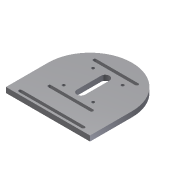
# Autodesk Inventor part: JointB1
Saved by Autodesk Inventor 2013 (Build 170138000, 138)
## iProperties
Created: 2012-10-15
Part Number: JointB1
Document SubType Name: Modeling
Designer: JohnHenry
Density: 1 g/cm^3
Mass: 25.0658 g
Surface Area: 135.276 cm^2
Volume: 25.0658 cm^3
Material: 一般
Author: JohnHenry
Autodesk Inventor part; units mm, degrees
ref_plane "YZ Plane" through (0, 0, 0) normal (1, 0, 0) x (0, 1, 0)
ref_plane "XZ Plane" through (0, 0, 0) normal (0, 1, 0) x (-1, 0, 0)
ref_plane "XY Plane" through (0, 0, 0) normal (0, 0, 1) x (1, 0, 0)
sketch "スケッチ1" plane through (0, 0, 0) normal (0, 0, 1) x (1, 0, 0)
  line L0 (-40, 67.6823) -> (40, 67.6823)
  line L1 (40, 67.6823) -> (40, -12.3177)
  line L2 (40, -12.3177) -> (-40, -12.3177)
  line L3 (-40, -12.3177) -> (-40, 67.6823)
  point P0 (0, 0)
  dimension "d0" = 80
  dimension "d1" = 40
  dimension "d2" = 80
  constraints: 8 end point, 2 parallel, 1 horizontal, 1 perpendicular
  measures "d0" distance of L1.end L2.end
  measures "d1" distance from line of L3 point (0, 0)
  measures "d2" distance of L2.end L0.start
extrude "押し出し1" add sketch "スケッチ1" along normal blind 5
sketch "スケッチ5" plane through (0, 0, 5) normal (0, 0, 1) x (1, 0, 0)
  line L0 (-40, -7.3177) -> (40, -7.3177) projected
  line L1 (40, 67.6823) -> (40, -12.3177) projected
  line L2 (-40, 67.6823) -> (40, 67.6823) projected
  line L3 (-40, -12.3177) -> (-40, 67.6823) projected
  arc A0 (40, 27.6823) -> (-40, 27.6823) centre (0, 27.6823) ccw
  point P0 (0, 0)
  dimension "d21" = 40
  dimension "d22" = 40
  dimension "d23" = 80
  constraints: 2 midpoint, 2 point on circle, 1 centre point, 1 coincident
  measures "d21" distance from line of point (0, 27.682) L2
  measures "d22" distance from line of L3 point (0, 27.682)
  measures "d23" diameter of A0
extrude "押し出し4" cut sketch "スケッチ5" against normal through all contours L3 L2 A0 | A0 L2 L1
sketch "スケッチ6" plane through (0, 0, 5) normal (0, 0, 1) x (1, 0, 0)
  arc A0 (40, 27.6823) -> (-40, 27.6823) centre (0, 27.6823) ccw projected
  point P0 (0, 0)
  constraints: 1 coincident
hole "Hole2" at (0, 27.6823, 5) direction (0, 0, -1) diameter 8 end through all
sketch "スケッチ8" plane through (0, 0, 5) normal (0, 0, 1) x (1, 0, 0)
  circle A0 centre (0, 27.6823) radius 4 projected
  line L0 (-20, 10.6823) -> (20, 10.6823)
  line L1 (20, 10.6823) -> (20, 7.6823)
  line L2 (20, 7.6823) -> (-20, 7.6823)
  line L3 (-20, 7.6823) -> (-20, 10.6823)
  circle A1 centre (-20, 9.1823) radius 1.5
  circle A2 centre (20, 9.1823) radius 1.5
  line L4 (40, -12.3177) -> (-40, -12.3177) projected
  line L5 (-20, 53.6823) -> (20, 53.6823)
  line L6 (20, 53.6823) -> (20, 50.6823)
  line L7 (20, 50.6823) -> (-20, 50.6823)
  line L8 (-20, 50.6823) -> (-20, 53.6823)
  circle A3 centre (-20, 52.1823) radius 1.5
  circle A4 centre (20, 52.1823) radius 1.5
  point P0 (0, 0)
  dimension "d54" = 3
  dimension "d55" = 20
  dimension "d56" = 40
  dimension "d65" = 20
  dimension "d87" = 40
  dimension "d88" = 20
  dimension "d89" = 3
  dimension "d91" = 40
  constraints: 16 end point, 4 midpoint, 4 parallel, 4 vertical alignment, 2 horizontal, 2 perpendicular, 8 other
  measures "d54" distance of L0.end L1.end
  measures "d55" distance from line of A0.centre L1
  measures "d56" distance of L1.end L2.end
  measures "d65" distance between parallel lines of L4 L2
  measures "d87" distance of L5.start L5.end
  measures "d88" distance from line of A0.centre L6
  measures "d89" distance of L5.end L6.end
  measures "d91" distance between parallel lines of L0 L7
extrude "押し出し5" cut sketch "スケッチ8" against normal through all contours A1 L3 | L0 A2 L2 A1 | L3 A1 | A2 L1 | L1 A2 | A3 L8 | L5 A4 L7 A3 | L8 A3 | A4 L6 | L6 A4
sketch "スケッチ9" plane through (0, 0, 5) normal (0, 0, 1) x (1, 0, 0)
  line L0 (-40, -12.3177) -> (-40, 27.6823) projected
  line L1 (40, -12.3177) -> (-40, -12.3177) projected
  line L2 (40, 27.6823) -> (40, -12.3177) projected
  line L3 (-30, -7.2177) -> (30, -7.2177)
  line L4 (30, -7.2177) -> (30, -10.2177)
  line L5 (30, -10.2177) -> (-30, -10.2177)
  line L6 (-30, -10.2177) -> (-30, -7.2177)
  circle A0 centre (-30, -8.7177) radius 1.5
  circle A1 centre (30, -8.7177) radius 1.5
  point P0 (0, 0)
  dimension "d59" = 3
  dimension "d60" = 10
  dimension "d61" = 10
  dimension "d62" = 5.1
  constraints: 8 end point, 2 midpoint, 2 parallel, 2 vertical alignment, 1 horizontal, 1 perpendicular, 4 other
  measures "d59" distance of L3.end L4.end
  measures "d60" distance between parallel lines of L2 L4
  measures "d61" distance between parallel lines of L0 L6
  measures "d62" distance between parallel lines of L1 L3
extrude "押し出し6" cut sketch "スケッチ9" against normal through all
sketch "スケッチ11" plane through (0, 0, 5) normal (0, 0, 1) x (1, 0, 0)
  arc A0 (20, 50.6823) -> (20, 53.6823) centre (20, 52.1823) ccw projected
  line L0 (20, 50.6823) -> (-20, 50.6823) projected
  line L1 (-20, 10.6823) -> (20, 10.6823) projected
  arc A1 (-20, 10.6823) -> (-20, 7.6823) centre (-20, 9.1823) ccw projected
  point P0 (0, 0)
  point P1 (-14, 44.6823)
  point P2 (-14, 16.6823)
  point P3 (14, 16.6823)
  point P4 (14, 44.6823)
  dimension "d92" = 6
  dimension "d93" = 6
  dimension "d94" = 6
  dimension "d95" = 6
  dimension "d96" = 6
  dimension "d97" = 6
  dimension "d98" = 6
  dimension "d99" = 6
  measures "d92" distance from line of point (-14, 44.682) L0
  measures "d93" horizontal distance of L0.end point (-14, 44.682)
  measures "d94" distance from line of L1 point (-14, 16.682)
  measures "d95" horizontal distance of point (-14, 16.682) A1.centre
  measures "d96" distance from line of L1 point (14, 16.682)
  measures "d97" horizontal distance of L1.end point (14, 16.682)
  measures "d98" horizontal distance of A0.centre point (14, 44.682)
  measures "d99" distance from line of point (14, 44.682) L0
hole "Hole5" at (-14, 44.6823, 5) at (-14, 16.6823, 5) at (14, 16.6823, 5) at (14, 44.6823, 5) direction (0, 0, -1) diameter 2.8 depth 8 tip angle 118
sketch "スケッチ12" plane through (0, 0, 5) normal (0, 0, 1) x (1, 0, 0)
  circle A0 centre (0, 27.6823) radius 4 projected
  line L0 (-4, 42.1823) -> (4, 42.1823)
  line L1 (4, 42.1823) -> (4, 19.1823)
  line L2 (4, 19.1823) -> (-4, 19.1823)
  line L3 (-4, 19.1823) -> (-4, 42.1823)
  circle A1 centre (0, 42.1823) radius 4
  circle A2 centre (0, 19.1823) radius 4
  circle A3 centre (14, 16.6823) radius 1.4 projected
  circle A4 centre (-14, 44.6823) radius 1.4 projected
  point P0 (0, 0)
  dimension "d109" = 2.5
  dimension "d110" = 2.5
  constraints: 8 end point, 2 horizontal alignment, 2 midpoint, 2 parallel, 1 horizontal, 1 perpendicular, 4 other
  measures "d109" distance from line of A3.centre L2
  measures "d110" distance from line of L0 A4.centre
extrude "押し出し7" cut sketch "スケッチ12" against normal blind 10 contours L1 A2 L3 A0 | A0 L3 A1 L1 | A1 L0 | L0 A1 | A2 L2 | L2 A2
equation "\"d1\" = 0.5 * d0"
equation "\"d2\" = d0"
equation "\"d21\" = d22"
equation "\"d55\" = 0.5 * d56"
equation "\"d87\" = d56"
equation "\"d88\" = d55"
equation "\"d89\" = d54"
equation "\"d61\" = d60"
equation "\"d93\" = d92"
equation "\"d94\" = d92"
equation "\"d95\" = d92"
equation "\"d96\" = d92"
equation "\"d97\" = d92"
equation "\"d98\" = d92"
equation "\"d99\" = d92"
equation "\"d110\" = d109"
